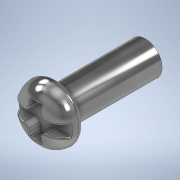
# Autodesk Inventor part: tamiya-slim-tire-bolt
Saved by Autodesk Inventor 2021 (Build 250183000, 183)
## iProperties
Created: 2023-10-14
Part Number: tamiya-slim-tire-bolt
Material: 一般
Document SubType Name: Modeling
Designer: takag
Density: 1 g/cm^3
Appearance: 鋼材 メッキ
Author: takag
Autodesk Inventor part; units mm, degrees
ref_plane "YZ Plane" through (0, 0, 0) normal (1, 0, 0) x (0, 1, 0)
ref_plane "XZ Plane" through (0, 0, 0) normal (0, 1, 0) x (-1, 0, 0)
ref_plane "XY Plane" through (0, 0, 0) normal (0, 0, 1) x (1, 0, 0)
sketch "スケッチ1" plane through (0, 0, 0) normal (0, 0, 1) x (1, 0, 0)
  circle A0 centre (0, 0) radius 1.5
  dimension "d0" = 3
  constraints: 1 centre point, 1 coincident
  measures "d0" diameter of A0
extrude "押し出し1" add sketch "スケッチ1" against normal blind 8
sketch "スケッチ2" plane through (0, 0, 0) normal (0, 1, 0) x (-1, 0, 0)
  line L0 (0, 0) -> (2.5, 0)
  line L1 (1.5, 0) -> (-1.5, 0) projected
  line L2 (0, 0) -> (-2.5, 0)
  line L3 (2.5, 0) -> (-2.5, 0)
  line L4 (-2.5, 0) -> (-2.5, 2)
  line L5 (-2.5, 2) -> (2.5, 2)
  line L6 (2.5, 2) -> (2.5, 0)
  line L7 (0, 2) -> (0, 0)
  dimension "d3" = 2.5
  dimension "d4" = 2.5
  dimension "d5" = 5
  dimension "d6" = 2
  constraints: 14 end point, 2 parallel, 1 collinear, 1 horizontal, 1 midpoint, 1 perpendicular, 1 point on line
  measures "d3" distance of L0.start L0.end
  measures "d4" distance of L0.start L2.end
  measures "d5" distance of L4.end L5.end
  measures "d6" distance of L3.end L4.end
revolve "回転1" add sketch "スケッチ2" angle 360 about axis through (0, 0, 2) along (0, 0, -1) contours L7 L5 L6 L0
fillet "フィレット1" radius 0.5 1 edges at (2.5, 0, 0)
fillet "フィレット2" radius 1.5 1 edges at (2.5, 0, 2)
sketch "スケッチ3" plane through (0, 0, 2) normal (0, 0, 1) x (1, 0, 0)
  line L0 (-2.5, 0.5) -> (2.5, 0.5)
  line L1 (2.5, 0.5) -> (2.5, -0.5)
  line L2 (2.5, -0.5) -> (-2.5, -0.5)
  line L3 (-2.5, -0.5) -> (-2.5, 0.5)
  line L4 (-2.5, 0.5) -> (2.5, -0.5) construction
  line L5 (2.5, 0.5) -> (-2.5, -0.5) construction
  point P0 (0, 0)
  dimension "d10" = 5
  dimension "d11" = 1
  constraints: 12 end point, 2 midpoint, 2 parallel, 1 horizontal, 1 perpendicular
  measures "d10" distance of L1.end L2.end
  measures "d11" distance of L0.end L1.end
extrude "押し出し2" cut sketch "スケッチ3" against normal blind 1
sketch "スケッチ4" plane through (0, 0, 2) normal (0, 0, 1) x (1, 0, 0)
  line L0 (-0.5, -1.5) -> (0.5, -1.5)
  line L1 (0.5, -1.5) -> (0.5, 1.5)
  line L2 (0.5, 1.5) -> (-0.5, 1.5)
  line L3 (-0.5, 1.5) -> (-0.5, -1.5)
  line L4 (-0.5, -1.5) -> (0.5, 1.5) construction
  line L5 (0.5, -1.5) -> (-0.5, 1.5) construction
  point P0 (0, 0)
  dimension "d14" = 1
  dimension "d15" = 3
  constraints: 12 end point, 2 midpoint, 2 parallel, 1 horizontal, 1 perpendicular
  measures "d14" distance of L2.end L1.end
  measures "d15" distance of L1.end L0.end
extrude "押し出し3" cut sketch "スケッチ4" against normal blind 1
fillet "フィレット3" radius 0.5 4 edges at (-0.5, 0.5, 1.5) (0.5, 0.5, 1.5) (-0.5, -0.5, 1.5) (0.5, -0.5, 1.5)
fillet "フィレット4" radius 0.1 4 edges at (-0.5, 1.5, 1.4415) (0.5, 1.5, 1.4415) (0.5, -1.5, 1.4415) (-0.5, -1.5, 1.4415)
fillet "フィレット5" radius 0.1 18 edges at (-1.8295, 0.5, 1.7028) (-0.6465, 0.6464, 1.9975) (-0.5, 1.2012, 1.9696) (-0.4707, 1.4707, 1.898) (0, 1.5, 1.9144) (0.4707, 1.4707, 1.898) (0.5, 1.2012, 1.9696) (0.6464, 0.6465, 1.9975) (1.8295, 0.5, 1.7028) (-0.6464, -0.6465, 1.9975) (-0.5, -1.2012, 1.9696) (-0.4707, -1.4707, 1.898) (0, -1.5, 1.9144) (0.4707, -1.4707, 1.898) (0.5, -1.2012, 1.9696) (0.6465, -0.6464, 1.9975) (1.8295, -0.5, 1.7028) (-1.8295, -0.5, 1.7028)
